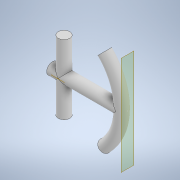
# Autodesk Inventor part: anchorPlaceholder
Saved by Autodesk Inventor 2021 (Build 250183000, 183)
## iProperties
Created: 2021-03-02
Part Number: anchorPlaceholder
Material: Generic
Document SubType Name: Modeling
Designer: con_c_000
Density: 1 g/cm^3
Appearance: Default
Author: con_c_000
## iProperties of the stored document _3DPrint.ipt
Created: 2021-03-02
Part Number: _3DPrint
Material: Generic
Document SubType Name: Modeling
Designer: con_c_000
Density: 1 g/cm^3
Appearance: Default
Author: con_c_000
Autodesk Inventor part; units mm, degrees
ref_plane "YZ Plane" through (0, 0, 0) normal (1, 0, 0) x (0, 1, 0)
ref_plane "XZ Plane" through (0, 0, 0) normal (0, 1, 0) x (-1, 0, 0)
ref_plane "XY Plane" through (0, 0, 0) normal (0, 0, 1) x (1, 0, 0)
sketch "Sketch1" plane through (0, 0, 0) normal (0, 1, 0) x (-1, 0, 0)
  circle A0 centre (0, 0) radius 12.7
  dimension "d0" = 25.4
  constraints: 1 centre point, 1 coincident
  measures "d0" diameter of A0
extrude "Extrusion1" add sketch "Sketch1" along normal blind 152.4
sketch "Sketch2" plane through (0, 0, 0) normal (1, 0, 0) x (0, 1, 0)
  circle A0 centre (76.2, 0) radius 12.7
  point P0 (0, 0)
  constraints: 1 centre point
extrude "Extrusion2" add sketch "Sketch2" along normal blind 127 and the other way blind 25.4
ref_plane "Work Plane1" through (0, 76.2, 0) normal (0, 1, 0) x (1, 0, 0)
sketch "Sketch3" plane through (0, 76.2, 0) normal (0, 1, 0) x (1, 0, 0)
  line L0 (127, -12.7) -> (127, 12.7) projected
  circle A0 centre (127, 0) radius 12.7
  line L1 (0, -22.5547) -> (0, 28.0783)
  point P0 (0, 0)
  constraints: 2 end point, 1 vertical, 1 vertical alignment, 2 other
revolve "Revolution1" add sketch "Sketch3" angle 90 mid plane about axis through (0, 76.2, 22.5547) along (0, 0, -1)
ref_plane "Work Plane3" through (139.7, 76.2, 12.7) normal (-1, 0, 0) x (0, 0, 1)
ref_plane "Work Plane2" through (127, 76.2, 12.7) normal (-1, 0, 0) x (0, 0, 1)
body "Solid1"
